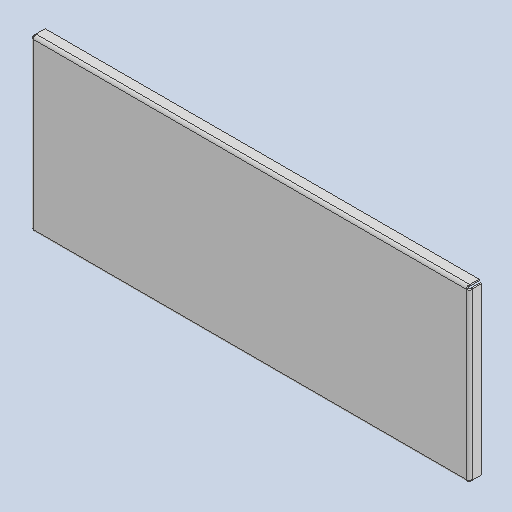
# Autodesk Inventor part: TapaDown
Saved by Autodesk Inventor 2023 (Build 270158000, 158)
## iProperties
Created: 2022-11-27
Part Number: TapaDown
Material: Generic
Document SubType Name: Sheet Metal
Designer: David
Density: 1 g/cm^3
Sheet Metal Rule: Default
Appearance: Default
Flat Pattern Width: 38.9405 cm
Flat Pattern Length: 93.9405 cm
Flat Pattern Area: 3658.09 cm^2
Sheet Metal Width: 389,405 mm
Sheet Metal Length: 939,405 mm
Sheet Metal Area: 365808,774 mm^2
Author: David
Autodesk Inventor part; units mm, degrees
note: some values were not read from the file. Chosen so that the rebuilt part matches the saved one: corner form of "Plate2".
ref_plane "YZ Plane" through (0, 0, 0) normal (1, 0, 0) x (0, 1, 0)
ref_plane "XZ Plane" through (0, 0, 0) normal (0, 1, 0) x (-1, 0, 0)
ref_plane "XY Plane" through (0, 0, 0) normal (0, 0, 1) x (1, 0, 0)
sketch "Sketch2" plane through (0, 0, 0) normal (0, 0, 1) x (1, 0, 0)
  line L0 (-450, -175) -> (450, -175)
  line L1 (450, -175) -> (450, 175)
  line L2 (450, 175) -> (-450, 175)
  line L3 (-450, 175) -> (-450, -175)
  line L4 (-450, -175) -> (450, 175) construction
  line L5 (450, -175) -> (-450, 175) construction
  point P0 (0, 0)
  dimension "d0" = 900
  dimension "d1" = 350
  measures "d0" distance of L2.end L1.end
  measures "d1" distance of L1.end L0.end
extrude "Plate1" add sketch "Sketch2" along normal mid plane 3.048
sketch "Sketch3" plane through (450, 171.952, 1.524) normal (0, 1, 0) x (-1, 0, 0)
  line L0 (900, 0) -> (0, 0)
  line L1 (0, 0) -> (0, -25)
  line L2 (0, -25) -> (900, -25)
  line L3 (900, -25) -> (900, 0)
  constraints: 6 end point, 1 horizontal, 1 perpendicular, 1 vertical
edge flange "Flange1" height 25 angle 90 thickness 3.048 bend radius 3.048 thickness toward (0, 1, 0) relief tear relief width 3.048 relief depth 1.524 corner gap 3.048 corner form 2 edges at (0, 175, -1.524) (-450, 0, -1.524) (0, -175, -1.524) (450, 0, -1.524) wall of the first edge with corners at (-450, 171.952, 1.524) (450, 171.952, 1.524) (450, 171.952, -23.476) (-450, 171.952, -23.476)
bend "Bend1"
corner "Corner1"
equation "\"d2\" = Thickness"
equation "\"d3\" = BendReliefWidth"
equation "\"d4\" = BendReliefDepth"
equation "\"d5\" = MinimumRemnant"
equation "\"d6\" = TransitionRadius"
equation "\"d9\" = BendRadius"
equation "\"d10\" = CornerReliefSize"
equation "\"d11\" = GapSize"
equation "\"d12\" = JacobiRadiusSize"
equation "\"BendRadius\" = Thickness"
equation "\"BendReliefWidth\" = Thickness"
equation "\"BendReliefDepth\" = 0.5 * Thickness"
equation "\"CornerReliefSize\" = 4 * Thickness"
equation "\"MinimumRemnant\" = 2 * Thickness"
equation "\"TransitionRadius\" = BendRadius"
equation "\"JacobiRadiusSize\" = BendRadius"
equation "\"GapSize\" = Thickness"
equation "\"Space5\" = 0"
equation "\"Space6\" = 0"
equation "\"Space7\" = 0"
equation "\"Thickness\" = 3.048"
body "Solid1"
